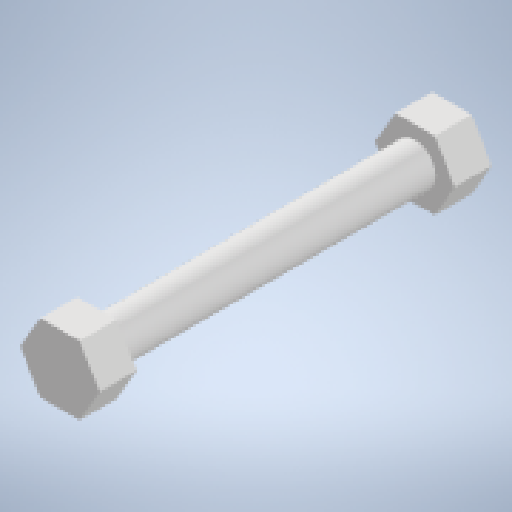
# Autodesk Inventor part: hing rod
Saved by Autodesk Inventor 2025.2 (Build 292293000, 293)
## iProperties
Created: 2025-01-08
Part Number: hing rod
Material: Generic
Document SubType Name: Modeling
Designer: 5013908
Density: 1 g/cm^3
Appearance: Default
Author: 5013908
Autodesk Inventor part; units mm, degrees
ref_plane "YZ Plane" through (0, 0, 0) normal (1, 0, 0) x (0, 1, 0)
ref_plane "XZ Plane" through (0, 0, 0) normal (0, 1, 0) x (-1, 0, 0)
ref_plane "XY Plane" through (0, 0, 0) normal (0, 0, 1) x (1, 0, 0)
sketch "Sketch1" plane through (0, 0, 0) normal (0, 0, 1) x (1, 0, 0)
  circle A0 centre (0, 0) radius 5
  circle A1 centre (0, 0) radius 9.5
  line L0 (-4.75, 8.2272) -> (4.75, 8.2272)
  line L1 (4.75, 8.2272) -> (9.5, 0)
  line L2 (9.5, 0) -> (4.75, -8.2272)
  line L3 (4.75, -8.2272) -> (-4.75, -8.2272)
  line L4 (-4.75, -8.2272) -> (-9.5, 0)
  line L5 (-9.5, 0) -> (-4.75, 8.2272)
  dimension "d0" = 10
  dimension "d1" = 19
  constraints: 12 end point, 6 point on circle, 3 equal length, 2 centre point, 2 coincident, 2 parallel, 1 horizontal
  measures "d0" diameter of A0
  measures "d1" diameter of A1
extrude "Extrusion1" add sketch "Sketch1" along normal blind 8.89 contours L2 L3 L4 L5 L0 L1
sketch "Sketch2" plane through (0, 0, 0) normal (0, 0, -1) x (-1, 0, 0)
  circle A0 centre (0, 0) radius 5
  dimension "d4" = 10
  constraints: 1 centre point, 1 coincident
  measures "d4" diameter of A0
extrude "Extrusion2" add sketch "Sketch2" against normal blind 94.0435
sketch "Sketch3" plane through (0, 0, 94.0435) normal (0, 0, 1) x (1, 0, 0)
  line L0 (-4.75, 8.2272) -> (-9.5, 0) projected
  circle A0 centre (0, 0) radius 9.5
  line L1 (-9.5, 0) -> (-4.75, 8.2272)
  line L2 (4.75, 8.2272) -> (-4.75, 8.2272) projected
  line L3 (-4.75, 8.2272) -> (4.75, 8.2272)
  line L4 (9.5, 0) -> (4.75, 8.2272) projected
  line L5 (4.75, 8.2272) -> (9.5, 0)
  line L6 (9.5, 0) -> (4.75, -8.2272)
  line L7 (4.75, -8.2272) -> (-4.75, -8.2272)
  line L8 (-4.75, -8.2272) -> (-9.5, 0)
  constraints: 12 end point, 6 equal length, 3 point on circle, 1 centre point, 1 coincident
extrude "Extrusion3" add sketch "Sketch3" against normal blind 8.89 contours L2 L4 L6 L7 L8 L0
body "Solid1"
